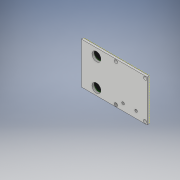
# Autodesk Inventor part: Печатная плата принимающая ось Z
Saved by Autodesk Inventor 2019 (Build 230136000, 136)
## iProperties
Created: 2019-08-27
Part Number: Печатная плата принимающая ось Z
Material: Типовые
Document SubType Name: Modeling
Designer: Петров Иван
Density: 1 g/cm^3
Appearance: По умолчанию
Autodesk Inventor part; units mm, degrees
(part 1 of 3)
ref_plane "YZ Plane" through (0, 0, 0) normal (1, 0, 0) x (0, 1, 0)
ref_plane "XZ Plane" through (0, 0, 0) normal (0, 1, 0) x (-1, 0, 0)
ref_plane "XY Plane" through (0, 0, 0) normal (0, 0, 1) x (1, 0, 0)
sketch "Эскиз1" plane through (0, 0, 0) normal (0, 0, 1) x (1, 0, 0)
  arc A0 (33.9725, 26.67) -> (33.3375, 26.67) centre (33.655, 26.67) ccw
  line L0 (27.051, 13.335) -> (30.988, 13.335)
  arc A1 (30.988, 13.0175) -> (30.988, 13.6525) centre (30.988, 13.335) ccw
  arc A2 (27.051, 13.6525) -> (27.051, 13.0175) centre (27.051, 13.335) ccw
  arc A3 (33.3375, 22.479) -> (33.9725, 22.479) centre (33.655, 22.479) ccw
  line L1 (33.655, 26.67) -> (33.655, 22.479)
  arc A4 (29.6525, 6.225) -> (30.2875, 6.225) centre (29.97, 6.225) ccw
  line L2 (29.97, 7.38) -> (29.97, 6.225)
  arc A5 (44.9285, 12.5435) -> (44.4795, 12.0945) centre (44.704, 12.319) ccw
  arc A6 (44.6575, 11.9165) -> (45.1065, 12.3655) centre (44.882, 12.141) ccw
  line L3 (44.704, 12.319) -> (44.882, 12.141)
  arc A7 (45.0215, 13.208) -> (44.3865, 13.208) centre (44.704, 13.208) ccw
  arc A8 (44.3865, 12.319) -> (45.0215, 12.319) centre (44.704, 12.319) ccw
  line L4 (44.704, 13.208) -> (44.704, 12.319)
  arc A9 (37.8165, 34.5145) -> (37.3675, 34.0655) centre (37.592, 34.29) ccw
  arc A10 (41.1775, 30.2555) -> (41.6265, 30.7045) centre (41.402, 30.48) ccw
  line L5 (37.592, 34.29) -> (41.402, 30.48)
  arc A11 (36.83, 34.6075) -> (36.83, 33.9725) centre (36.83, 34.29) ccw
  arc A12 (37.592, 33.9725) -> (37.592, 34.6075) centre (37.592, 34.29) ccw
  line L6 (36.83, 34.29) -> (37.592, 34.29)
  arc A13 (32.3555, 34.0655) -> (31.9065, 34.5145) centre (32.131, 34.29) ccw
  arc A14 (29.3665, 31.9745) -> (29.8155, 31.5255) centre (29.591, 31.75) ccw
  line L7 (32.131, 34.29) -> (29.591, 31.75)
  arc A15 (36.83, 33.9725) -> (36.83, 34.6075) centre (36.83, 34.29) ccw
  arc A16 (32.131, 34.6075) -> (32.131, 33.9725) centre (32.131, 34.29) ccw
  line L8 (36.83, 34.29) -> (32.131, 34.29)
  arc A17 (29.591, 31.4325) -> (29.591, 32.0675) centre (29.591, 31.75) ccw
  arc A18 (26.67, 32.0675) -> (26.67, 31.4325) centre (26.67, 31.75) ccw
  line L9 (29.591, 31.75) -> (26.67, 31.75)
  arc A19 (40.4155, 22.1955) -> (40.8645, 21.7465) centre (40.64, 21.971) ccw
  arc A20 (41.6265, 22.5085) -> (41.1775, 22.9575) centre (41.402, 22.733) ccw
  line L10 (40.64, 21.971) -> (41.402, 22.733)
  arc A21 (41.7195, 22.733) -> (41.0845, 22.733) centre (41.402, 22.733) ccw
  line L11 (26.289, 14.097) -> (27.051, 13.335)
  arc A22 (24.638, 24.8285) -> (24.638, 24.1935) centre (24.638, 24.511) ccw
  arc A23 (38.1, 24.1935) -> (38.1, 24.8285) centre (38.1, 24.511) ccw
  line L12 (24.638, 24.511) -> (38.1, 24.511)
  arc A24 (22.0005, 22.3225) -> (22.4495, 21.8735) centre (22.225, 22.098) ccw
  arc A25 (24.8625, 24.2865) -> (24.4135, 24.7355) centre (24.638, 24.511) ccw
  line L13 (22.225, 22.098) -> (24.638, 24.511)
  arc A26 (21.0185, 20.574) -> (20.3835, 20.574) centre (20.701, 20.574) ccw
  arc A27 (20.3835, 15.24) -> (21.0185, 15.24) centre (20.701, 15.24) ccw
  line L14 (20.701, 20.574) -> (20.701, 15.24)
  arc A28 (22.4495, 21.8735) -> (22.0005, 22.3225) centre (22.225, 22.098) ccw
  arc A29 (20.4765, 20.7985) -> (20.9255, 20.3495) centre (20.701, 20.574) ccw
  line L15 (22.225, 22.098) -> (20.701, 20.574)
  line L16 (22.225, 19.558) -> (26.035, 16.637)
  arc A30 (19.0205, 12.9245) -> (18.5715, 12.4755) centre (18.796, 12.7) ccw
  arc A31 (20.0955, 10.9515) -> (20.5445, 11.4005) centre (20.32, 11.176) ccw
  line L17 (18.796, 12.7) -> (20.32, 11.176)
  arc A32 (19.1135, 21.971) -> (18.4785, 21.971) centre (18.796, 21.971) ccw
  arc A33 (18.4785, 12.7) -> (19.1135, 12.7) centre (18.796, 12.7) ccw
  line L18 (18.796, 21.971) -> (18.796, 12.7)
  arc A34 (20.32, 11.3665) -> (20.32, 10.7315) centre (20.32, 11.049) ccw
  arc A35 (24.261, 10.7315) -> (24.261, 11.3665) centre (24.261, 11.049) ccw
  line L19 (20.32, 11.049) -> (24.261, 11.049)
  arc A36 (27.7055, 7.1555) -> (28.1545, 7.6045) centre (27.93, 7.38) ccw
  arc A37 (24.4855, 11.2735) -> (24.0365, 10.8245) centre (24.261, 11.049) ccw
  line L20 (27.93, 7.38) -> (24.261, 11.049)
  arc A38 (33.9725, 22.479) -> (33.3375, 22.479) centre (33.655, 22.479) ccw
  arc A39 (33.3375, 19.304) -> (33.9725, 19.304) centre (33.655, 19.304) ccw
  line L21 (33.655, 22.479) -> (33.655, 19.304)
  arc A40 (21.59, 26.9875) -> (21.59, 26.3525) centre (21.59, 26.67) ccw
  arc A41 (33.655, 26.3525) -> (33.655, 26.9875) centre (33.655, 26.67) ccw
  line L22 (21.59, 26.67) -> (33.655, 26.67)
  arc A42 (21.59, 26.3525) -> (20.955, 26.3525) centre (21.2725, 26.3525) ccw
  arc A43 (20.955, 24.4475) -> (21.59, 24.4475) centre (21.2725, 24.4475) ccw
  line L23 (21.2725, 26.3525) -> (21.2725, 24.4475)
  arc A44 (21.8145, 26.4455) -> (21.3655, 26.8945) centre (21.59, 26.67) ccw
  arc A45 (21.048, 26.577) -> (21.497, 26.128) centre (21.2725, 26.3525) ccw
  line L24 (21.59, 26.67) -> (21.2725, 26.3525)
  arc A46 (18.5715, 22.1955) -> (19.0205, 21.7465) centre (18.796, 21.971) ccw
  arc A47 (21.497, 24.223) -> (21.048, 24.672) centre (21.2725, 24.4475) ccw
  line L25 (18.796, 21.971) -> (21.2725, 24.4475)
  arc A48 (37.7485, 19.5285) -> (38.1975, 19.0795) centre (37.973, 19.304) ccw
  arc A49 (38.3245, 19.2065) -> (37.8755, 19.6555) centre (38.1, 19.431) ccw
  line L26 (37.973, 19.304) -> (38.1, 19.431)
  arc A50 (33.655, 19.6215) -> (33.655, 18.9865) centre (33.655, 19.304) ccw
  arc A51 (41.0845, 21.209) -> (41.7195, 21.209) centre (41.402, 21.209) ccw
  line L27 (41.402, 22.733) -> (41.402, 21.209)
  arc A52 (41.7195, 30.48) -> (41.0845, 30.48) centre (41.402, 30.48) ccw
  arc A53 (41.0845, 22.733) -> (41.7195, 22.733) centre (41.402, 22.733) ccw
  line L28 (41.402, 30.48) -> (41.402, 22.733)
  arc A54 (41.6265, 15.9725) -> (41.1775, 15.5235) centre (41.402, 15.748) ccw
  arc A55 (41.6855, 15.0155) -> (42.1345, 15.4645) centre (41.91, 15.24) ccw
  line L29 (41.402, 15.748) -> (41.91, 15.24)
  arc A56 (41.7195, 15.875) -> (41.0845, 15.875) centre (41.402, 15.875) ccw
  arc A57 (41.0845, 15.748) -> (41.7195, 15.748) centre (41.402, 15.748) ccw
  line L30 (41.402, 15.875) -> (41.402, 15.748)
  arc A58 (41.6265, 15.6505) -> (41.1775, 16.0995) centre (41.402, 15.875) ccw
  arc A59 (40.5425, 15.4645) -> (40.9915, 15.0155) centre (40.767, 15.24) ccw
  line L31 (41.402, 15.875) -> (40.767, 15.24)
  arc A60 (41.7195, 21.209) -> (41.0845, 21.209) centre (41.402, 21.209) ccw
  arc A61 (41.0845, 15.875) -> (41.7195, 15.875) centre (41.402, 15.875) ccw
  line L32 (41.402, 21.209) -> (41.402, 15.875)
  arc A62 (40.8645, 22.1955) -> (40.4155, 21.7465) centre (40.64, 21.971) ccw
  arc A63 (41.1775, 20.9845) -> (41.6265, 21.4335) centre (41.402, 21.209) ccw
  line L33 (40.64, 21.971) -> (41.402, 21.209)
  arc A64 (38.1, 22.2885) -> (38.1, 21.6535) centre (38.1, 21.971) ccw
  arc A65 (40.64, 21.6535) -> (40.64, 22.2885) centre (40.64, 21.971) ccw
  line L34 (38.1, 21.971) -> (40.64, 21.971)
  arc A66 (42.8965, 15.4645) -> (42.4475, 15.0155) centre (42.672, 15.24) ccw
  arc A67 (44.4795, 12.9835) -> (44.9285, 13.4325) centre (44.704, 13.208) ccw
  line L35 (42.672, 15.24) -> (44.704, 13.208)
  arc A68 (41.91, 15.5575) -> (41.91, 14.9225) centre (41.91, 15.24) ccw
  arc A69 (42.672, 14.9225) -> (42.672, 15.5575) centre (42.672, 15.24) ccw
  line L36 (41.91, 15.24) -> (42.672, 15.24)
  arc A70 (40.767, 15.5575) -> (40.767, 14.9225) centre (40.767, 15.24) ccw
  arc A71 (41.91, 14.9225) -> (41.91, 15.5575) centre (41.91, 15.24) ccw
  line L37 (40.767, 15.24) -> (41.91, 15.24)
  arc A72 (35.052, 15.5575) -> (35.052, 14.9225) centre (35.052, 15.24) ccw
  arc A73 (40.767, 14.9225) -> (40.767, 15.5575) centre (40.767, 15.24) ccw
  line L38 (35.052, 15.24) -> (40.767, 15.24)
  arc A74 (33.8795, 16.8615) -> (33.4305, 16.4125) centre (33.655, 16.637) ccw
  arc A75 (34.8275, 15.0155) -> (35.2765, 15.4645) centre (35.052, 15.24) ccw
  line L39 (33.655, 16.637) -> (35.052, 15.24)
  arc A76 (31.623, 16.9545) -> (31.623, 16.3195) centre (31.623, 16.637) ccw
  arc A77 (33.655, 16.3195) -> (33.655, 16.9545) centre (33.655, 16.637) ccw
  line L40 (31.623, 16.637) -> (33.655, 16.637)
  arc A78 (31.2125, 17.4965) -> (30.7635, 17.0475) centre (30.988, 17.272) ccw
  arc A79 (31.3985, 16.4125) -> (31.8475, 16.8615) centre (31.623, 16.637) ccw
  line L41 (30.988, 17.272) -> (31.623, 16.637)
  arc A80 (31.3055, 17.399) -> (30.6705, 17.399) centre (30.988, 17.399) ccw
  arc A81 (30.6705, 17.272) -> (31.3055, 17.272) centre (30.988, 17.272) ccw
  line L42 (30.988, 17.399) -> (30.988, 17.272)
  arc A82 (29.4345, 19.4015) -> (28.9855, 18.9525) centre (29.21, 19.177) ccw
  arc A83 (30.7635, 17.1745) -> (31.2125, 17.6235) centre (30.988, 17.399) ccw
  line L43 (29.21, 19.177) -> (30.988, 17.399)
  arc A84 (37.0005, 10.1445) -> (37.4495, 9.6955) centre (37.225, 9.92) ccw
  arc A85 (26.162, 19.4945) -> (26.162, 18.8595) centre (26.162, 19.177) ccw
  arc A86 (29.21, 18.8595) -> (29.21, 19.4945) centre (29.21, 19.177) ccw
  line L44 (26.162, 19.177) -> (29.21, 19.177)
  arc A87 (26.2595, 19.5285) -> (25.8105, 19.0795) centre (26.035, 19.304) ccw
  arc A88 (25.9375, 18.9525) -> (26.3865, 19.4015) centre (26.162, 19.177) ccw
  line L45 (26.035, 19.304) -> (26.162, 19.177)
  arc A89 (27.5175, 16.8615) -> (27.0685, 16.4125) centre (27.293, 16.637) ccw
  arc A90 (28.7255, 14.7555) -> (29.1745, 15.2045) centre (28.95, 14.98) ccw
  line L46 (27.293, 16.637) -> (28.95, 14.98)
  arc A91 (26.035, 16.9545) -> (26.035, 16.3195) centre (26.035, 16.637) ccw
  arc A92 (27.293, 16.3195) -> (27.293, 16.9545) centre (27.293, 16.637) ccw
  line L47 (26.035, 16.637) -> (27.293, 16.637)
  arc A93 (29.2675, 14.98) -> (28.6325, 14.98) centre (28.95, 14.98) ccw
  arc A94 (28.6325, 9.92) -> (29.2675, 9.92) centre (28.95, 9.92) ccw
  line L48 (28.95, 14.98) -> (28.95, 9.92)
  arc A95 (24.892, 22.5425) -> (24.892, 21.9075) centre (24.892, 22.225) ccw
  arc A96 (30.988, 21.9075) -> (30.988, 22.5425) centre (30.988, 22.225) ccw
  line L49 (24.892, 22.225) -> (30.988, 22.225)
  arc A97 (22.0005, 19.7825) -> (22.4495, 19.3335) centre (22.225, 19.558) ccw
  arc A98 (25.1165, 22.0005) -> (24.6675, 22.4495) centre (24.892, 22.225) ccw
  line L50 (22.225, 19.558) -> (24.892, 22.225)
  arc A99 (22.4182, 19.81) -> (22.0318, 19.306) centre (22.225, 19.558) ccw
  arc A100 (25.8418, 16.385) -> (26.2282, 16.889) centre (26.035, 16.637) ccw
  arc A101 (20.6375, 11.176) -> (20.0025, 11.176) centre (20.32, 11.176) ccw
  arc A102 (20.0025, 11.049) -> (20.6375, 11.049) centre (20.32, 11.049) ccw
  line L51 (20.32, 11.176) -> (20.32, 11.049)
  arc A103 (37.973, 18.9865) -> (37.973, 19.6215) centre (37.973, 19.304) ccw
  line L52 (33.655, 19.304) -> (37.973, 19.304)
  arc A104 (39.878, 7.8105) -> (39.878, 8.4455) centre (39.878, 8.128) ccw
  arc A105 (32.758, 8.4455) -> (32.758, 7.8105) centre (32.758, 8.128) ccw
  line L53 (39.878, 8.128) -> (32.758, 8.128)
  arc A106 (42.1345, 9.9355) -> (41.6855, 10.3845) centre (41.91, 10.16) ccw
  arc A107 (39.6535, 8.3525) -> (40.1025, 7.9035) centre (39.878, 8.128) ccw
  line L54 (41.91, 10.16) -> (39.878, 8.128)
  arc A108 (42.2275, 12.065) -> (41.5925, 12.065) centre (41.91, 12.065) ccw
  arc A109 (41.5925, 10.16) -> (42.2275, 10.16) centre (41.91, 10.16) ccw
  line L55 (41.91, 12.065) -> (41.91, 10.16)
  arc A110 (42.3885, 12.0945) -> (41.9395, 12.5435) centre (42.164, 12.319) ccw
  arc A111 (41.6855, 12.2895) -> (42.1345, 11.8405) centre (41.91, 12.065) ccw
  line L56 (42.164, 12.319) -> (41.91, 12.065)
  arc A112 (32.9825, 7.9035) -> (32.5335, 8.3525) centre (32.758, 8.128) ccw
  arc A113 (31.7855, 7.6045) -> (32.2345, 7.1555) centre (32.01, 7.38) ccw
  line L57 (32.758, 8.128) -> (32.01, 7.38)
  arc A114 (31.2125, 10.1465) -> (30.7635, 9.6975) centre (30.988, 9.922) ccw
  arc A115 (30.7655, 9.6955) -> (31.2145, 10.1445) centre (30.99, 9.92) ccw
  line L58 (30.988, 9.922) -> (30.99, 9.92)
  arc A116 (31.3055, 13.335) -> (30.6705, 13.335) centre (30.988, 13.335) ccw
  arc A117 (30.6705, 9.922) -> (31.3055, 9.922) centre (30.988, 9.922) ccw
  line L59 (30.988, 13.335) -> (30.988, 9.922)
  arc A118 (21.844, 14.4145) -> (21.844, 13.7795) centre (21.844, 14.097) ccw
  arc A119 (26.289, 13.7795) -> (26.289, 14.4145) centre (26.289, 14.097) ccw
  line L60 (21.844, 14.097) -> (26.289, 14.097)
  arc A120 (20.9255, 15.4645) -> (20.4765, 15.0155) centre (20.701, 15.24) ccw
  arc A121 (21.6195, 13.8725) -> (22.0685, 14.3215) centre (21.844, 14.097) ccw
  line L61 (20.701, 15.24) -> (21.844, 14.097)
  arc A122 (26.5135, 14.3215) -> (26.0645, 13.8725) centre (26.289, 14.097) ccw
  arc A123 (26.8265, 13.1105) -> (27.2755, 13.5595) centre (27.051, 13.335) ccw
  arc A124 (39.8485, 12.0945) -> (39.3995, 12.5435) centre (39.624, 12.319) ccw
  line L62 (37.225, 9.92) -> (39.624, 12.319)
  arc A125 (33.03, 10.2375) -> (33.03, 9.6025) centre (33.03, 9.92) ccw
  arc A126 (37.225, 9.6025) -> (37.225, 10.2375) centre (37.225, 9.92) ccw
  line L63 (33.03, 9.92) -> (37.225, 9.92)
  arc A127 (21.59, 34.6075) -> (21.59, 33.9725) centre (21.59, 34.29) ccw
  arc A128 (26.67, 33.9725) -> (26.67, 34.6075) centre (26.67, 34.29) ccw
  line L64 (21.59, 34.29) -> (26.67, 34.29)
  arc A129 (34.7005, 30.0695) -> (35.1495, 29.6205) centre (34.925, 29.845) ccw
  arc A130 (37.0545, 31.5255) -> (36.6055, 31.9745) centre (36.83, 31.75) ccw
  line L65 (34.925, 29.845) -> (36.83, 31.75)
  arc A131 (30.988, 30.1625) -> (30.988, 29.5275) centre (30.988, 29.845) ccw
  arc A132 (34.925, 29.5275) -> (34.925, 30.1625) centre (34.925, 29.845) ccw
  line L66 (30.988, 29.845) -> (34.925, 29.845)
  arc A133 (45.1065, 7.1925) -> (44.6575, 7.6415) centre (44.882, 7.417) ccw
  arc A134 (39.4895, 2.4735) -> (39.9385, 2.0245) centre (39.714, 2.249) ccw
  line L67 (44.882, 7.417) -> (39.714, 2.249)
  arc A135 (45.1995, 12.141) -> (44.5645, 12.141) centre (44.882, 12.141) ccw
  arc A136 (44.5645, 7.417) -> (45.1995, 7.417) centre (44.882, 7.417) ccw
  line L68 (44.882, 12.141) -> (44.882, 7.417)
  arc A137 (30.1945, 6.4495) -> (29.7455, 6.0005) centre (29.97, 6.225) ccw
  arc A138 (33.7215, 2.0245) -> (34.1705, 2.4735) centre (33.946, 2.249) ccw
  line L69 (29.97, 6.225) -> (33.946, 2.249)
  arc A139 (39.714, 1.9315) -> (39.714, 2.5665) centre (39.714, 2.249) ccw
  arc A140 (33.946, 2.5665) -> (33.946, 1.9315) centre (33.946, 2.249) ccw
  line L70 (39.714, 2.249) -> (33.946, 2.249)
  arc A141 (30.2875, 7.38) -> (29.6525, 7.38) centre (29.97, 7.38) ccw
  line L71 (46.533, -1.143) -> (46.533, 36.947)
  line L72 (46.533, 36.947) -> (-13.871, 36.947)
  line L73 (-13.871, 36.947) -> (-13.871, -1.143)
  circle A142 centre (17.907, 34.925) radius 1.5
  circle A143 centre (17.907, 0.762) radius 1.5
  circle A144 centre (44.577, 0.762) radius 1.5
  circle A145 centre (44.704, 35.052) radius 1.5
  circle A146 centre (0, 30) radius 4.1
  circle A147 centre (0, 5) radius 4.1
  circle A148 centre (24.48, 5.08) radius 1.18
  line L74 (-13.871, -1.143) -> (46.533, -1.143)
  circle A149 centre (36.48, 5.08) radius 1.18
  arc A150 (39.8159, 21.3614) -> (39.8159, 21.4122) centre (39.8159, 21.3868) ccw
  arc A151 (39.1668, 21.6464) -> (39.4264, 21.3868) centre (39.4264, 21.6464) ccw
  arc A152 (39.1922, 21.6464) -> (39.1414, 21.6464) centre (39.1668, 21.6464) ccw
  arc A153 (39.4264, 21.3614) -> (39.4264, 21.4122) centre (39.4264, 21.3868) ccw
  line L75 (39.1668, 21.6464) -> (39.1668, 22.2956)
  arc A154 (39.1922, 22.2956) -> (39.1414, 22.2956) centre (39.1668, 22.2956) ccw
  arc A155 (39.1414, 21.6464) -> (39.1922, 21.6464) centre (39.1668, 21.6464) ccw
  arc A156 (39.4264, 22.5552) -> (39.1668, 22.2956) centre (39.4264, 22.2956) ccw
  arc A157 (39.4264, 22.5298) -> (39.4264, 22.5806) centre (39.4264, 22.5552) ccw
  arc A158 (39.1414, 22.2956) -> (39.1922, 22.2956) centre (39.1668, 22.2956) ccw
  line L76 (24.765, 30.48) -> (28.575, 30.48)
  arc A159 (28.575, 30.4292) -> (28.575, 30.5308) centre (28.575, 30.48) ccw
  arc A160 (24.765, 30.5308) -> (24.765, 30.4292) centre (24.765, 30.48) ccw
  arc A161 (28.575, 30.48) -> (24.765, 30.48) centre (26.67, 33.02) ccw
  line L77 (39.4264, 22.5552) -> (39.8159, 22.5552)
  arc A162 (39.8159, 22.5298) -> (39.8159, 22.5806) centre (39.8159, 22.5552) ccw
  arc A163 (39.4264, 22.5806) -> (39.4264, 22.5298) centre (39.4264, 22.5552) ccw
  line L78 (40.386, 21.3868) -> (40.386, 22.5552)
  arc A164 (40.4114, 22.5552) -> (40.3606, 22.5552) centre (40.386, 22.5552) ccw
  arc A165 (40.3606, 21.3868) -> (40.4114, 21.3868) centre (40.386, 21.3868) ccw
  line L79 (40.386, 22.5552) -> (41.0351, 21.3868)
  arc A166 (41.0129, 21.3745) -> (41.0573, 21.3991) centre (41.0351, 21.3868) ccw
  arc A167 (40.4082, 22.5675) -> (40.3638, 22.5429) centre (40.386, 22.5552) ccw
  line L80 (41.0351, 21.3868) -> (41.0351, 22.5552)
  arc A168 (41.0605, 22.5552) -> (41.0097, 22.5552) centre (41.0351, 22.5552) ccw
  arc A169 (41.0097, 21.3868) -> (41.0605, 21.3868) centre (41.0351, 21.3868) ccw
  line L81 (41.6052, 21.3868) -> (41.6052, 22.5552)
  arc A170 (41.6306, 22.5552) -> (41.5798, 22.5552) centre (41.6052, 22.5552) ccw
  arc A171 (41.5798, 21.3868) -> (41.6306, 21.3868) centre (41.6052, 21.3868) ccw
  line L82 (41.6052, 22.5552) -> (41.9297, 22.5552)
  arc A172 (41.9297, 22.5298) -> (41.9297, 22.5806) centre (41.9297, 22.5552) ccw
  arc A173 (41.6052, 22.5806) -> (41.6052, 22.5298) centre (41.6052, 22.5552) ccw
  arc A174 (42.2543, 22.2306) -> (41.9297, 22.5552) centre (41.9297, 22.2306) ccw
  arc A175 (42.2289, 22.2306) -> (42.2797, 22.2306) centre (42.2543, 22.2306) ccw
  arc A176 (41.9297, 22.5806) -> (41.9297, 22.5298) centre (41.9297, 22.5552) ccw
  line L83 (42.2543, 22.2306) -> (42.2543, 21.7114)
  arc A177 (42.2289, 21.7114) -> (42.2797, 21.7114) centre (42.2543, 21.7114) ccw
  arc A178 (42.2797, 22.2306) -> (42.2289, 22.2306) centre (42.2543, 22.2306) ccw
  arc A179 (41.9297, 21.3868) -> (42.2543, 21.7114) centre (41.9297, 21.7114) ccw
  arc A180 (41.9297, 21.4122) -> (41.9297, 21.3614) centre (41.9297, 21.3868) ccw
  arc A181 (42.2797, 21.7114) -> (42.2289, 21.7114) centre (42.2543, 21.7114) ccw
  line L84 (41.9297, 21.3868) -> (41.6052, 21.3868)
  arc A182 (41.6052, 21.4122) -> (41.6052, 21.3614) centre (41.6052, 21.3868) ccw
  arc A183 (41.9297, 21.3614) -> (41.9297, 21.4122) centre (41.9297, 21.3868) ccw
  arc A184 (26.67, 30.48) -> (26.67, 35.56) centre (26.67, 33.02) ccw
  arc A185 (26.67, 35.56) -> (26.67, 30.48) centre (26.67, 33.02) ccw
  line L85 (39.2938, 18.8468) -> (39.2938, 20.0152)
  arc A186 (39.3192, 20.0152) -> (39.2684, 20.0152) centre (39.2938, 20.0152) ccw
  arc A187 (39.2684, 18.8468) -> (39.3192, 18.8468) centre (39.2938, 18.8468) ccw
  line L86 (39.2938, 20.0152) -> (39.6184, 20.0152)
  arc A188 (39.6184, 19.9898) -> (39.6184, 20.0406) centre (39.6184, 20.0152) ccw
  arc A189 (39.2938, 20.0406) -> (39.2938, 19.9898) centre (39.2938, 20.0152) ccw
  arc A190 (39.9429, 19.6906) -> (39.6184, 20.0152) centre (39.6183, 19.6906) ccw
  arc A191 (39.9175, 19.6906) -> (39.9683, 19.6906) centre (39.9429, 19.6906) ccw
  arc A192 (39.6184, 20.0406) -> (39.6184, 19.9898) centre (39.6184, 20.0152) ccw
  line L87 (39.9429, 19.6906) -> (39.9429, 19.1714)
  line L88 (38.735, 35.56) -> (34.925, 35.56)
  arc A193 (34.925, 35.6108) -> (34.925, 35.5092) centre (34.925, 35.56) ccw
  arc A194 (38.735, 35.5092) -> (38.735, 35.6108) centre (38.735, 35.56) ccw
  arc A195 (34.925, 35.56) -> (38.735, 35.56) centre (36.83, 33.02) ccw
  arc A196 (39.9175, 19.1714) -> (39.9683, 19.1714) centre (39.9429, 19.1714) ccw
  arc A197 (39.9683, 19.6906) -> (39.9175, 19.6906) centre (39.9429, 19.6906) ccw
  arc A198 (39.6184, 18.8468) -> (39.9429, 19.1714) centre (39.6183, 19.1714) ccw
  arc A199 (39.6184, 18.8722) -> (39.6184, 18.8214) centre (39.6184, 18.8468) ccw
  arc A200 (39.9683, 19.1714) -> (39.9175, 19.1714) centre (39.9429, 19.1714) ccw
  line L89 (39.6184, 18.8468) -> (39.2938, 18.8468)
  arc A201 (39.2938, 18.8722) -> (39.2938, 18.8214) centre (39.2938, 18.8468) ccw
  arc A202 (39.6184, 18.8214) -> (39.6184, 18.8722) centre (39.6184, 18.8468) ccw
  line L90 (40.4749, 19.1714) -> (40.4749, 19.6906)
  arc A203 (40.5003, 19.6906) -> (40.4495, 19.6906) centre (40.4749, 19.6906) ccw
  arc A204 (41.124, 19.6906) -> (40.4749, 19.6906) centre (40.7995, 19.6906) ccw
  arc A205 (41.0986, 19.6906) -> (41.1494, 19.6906) centre (41.124, 19.6906) ccw
  arc A206 (40.4495, 19.6906) -> (40.5003, 19.6906) centre (40.4749, 19.6906) ccw
  line L91 (41.124, 19.6906) -> (41.124, 19.1714)
  arc A207 (41.0986, 19.1714) -> (41.1494, 19.1714) centre (41.124, 19.1714) ccw
  arc A208 (41.1494, 19.6906) -> (41.0986, 19.6906) centre (41.124, 19.6906) ccw
  arc A209 (40.4749, 19.1714) -> (41.124, 19.1714) centre (40.7995, 19.1714) ccw
  arc A210 (40.5003, 19.1714) -> (40.4495, 19.1714) centre (40.4749, 19.1714) ccw
  arc A211 (41.1494, 19.1714) -> (41.0986, 19.1714) centre (41.124, 19.1714) ccw
  line L92 (39.2938, 16.5608) -> (39.6833, 17.7292)
  arc A212 (39.7074, 17.7212) -> (39.6592, 17.7372) centre (39.6833, 17.7292) ccw
  arc A213 (39.2697, 16.5688) -> (39.3179, 16.5528) centre (39.2938, 16.5608) ccw
  line L93 (39.6833, 17.7292) -> (40.0727, 16.5608)
  arc A214 (40.0486, 16.5528) -> (40.0968, 16.5688) centre (40.0727, 16.5608) ccw
  arc A215 (39.7074, 17.7372) -> (39.6592, 17.7212) centre (39.6833, 17.7292) ccw
  line L94 (39.9754, 16.8529) -> (39.3912, 16.8529)
  arc A216 (39.3912, 16.8783) -> (39.3912, 16.8275) centre (39.3912, 16.8529) ccw
  arc A217 (39.9754, 16.8275) -> (39.9754, 16.8783) centre (39.9754, 16.8529) ccw
  line L95 (40.5017, 16.8854) -> (40.5017, 17.4046)
  arc A218 (40.5271, 17.4046) -> (40.4763, 17.4046) centre (40.5017, 17.4046) ccw
  arc A219 (40.4763, 16.8854) -> (40.5271, 16.8854) centre (40.5017, 16.8854) ccw
  arc A220 (41.1508, 17.4046) -> (40.5017, 17.4046) centre (40.8263, 17.4046) ccw
  arc A221 (41.1254, 17.4046) -> (41.1762, 17.4046) centre (41.1508, 17.4046) ccw
  arc A222 (40.4763, 17.4046) -> (40.5271, 17.4046) centre (40.5017, 17.4046) ccw
  line L96 (41.1508, 17.4046) -> (41.1508, 16.8854)
  arc A223 (41.1254, 16.8854) -> (41.1762, 16.8854) centre (41.1508, 16.8854) ccw
  arc A224 (36.83, 30.48) -> (36.83, 35.56) centre (36.83, 33.02) ccw
  arc A225 (36.83, 35.56) -> (36.83, 30.48) centre (36.83, 33.02) ccw
  arc A226 (41.1762, 17.4046) -> (41.1254, 17.4046) centre (41.1508, 17.4046) ccw
  line L97 (45.974, 13.589) -> (45.974, 11.684)
  arc A227 (45.9423, 11.684) -> (46.0058, 11.684) centre (45.9741, 11.684) ccw
  arc A228 (46.0058, 13.589) -> (45.9423, 13.589) centre (45.9741, 13.589) ccw
  line L98 (45.974, 11.684) -> (45.339, 11.049)
  arc A229 (45.3165, 11.0715) -> (45.3615, 11.0265) centre (45.339, 11.049) ccw
  arc A230 (45.9965, 11.6615) -> (45.9515, 11.7065) centre (45.974, 11.684) ccw
  line L99 (45.339, 11.049) -> (44.069, 11.049)
  arc A231 (44.069, 11.0808) -> (44.069, 11.0173) centre (44.069, 11.0491) ccw
  arc A232 (45.339, 11.0173) -> (45.339, 11.0808) centre (45.339, 11.0491) ccw
  line L100 (44.069, 11.049) -> (43.434, 11.684)
  arc A233 (43.4565, 11.7065) -> (43.4115, 11.6615) centre (43.434, 11.684) ccw
  arc A234 (44.0465, 11.0265) -> (44.0915, 11.0715) centre (44.069, 11.049) ccw
  line L101 (43.434, 11.684) -> (42.799, 11.049)
  arc A235 (42.7765, 11.0715) -> (42.8215, 11.0265) centre (42.799, 11.049) ccw
  arc A236 (43.4565, 11.6615) -> (43.4115, 11.7065) centre (43.434, 11.684) ccw
  line L102 (42.799, 11.049) -> (41.529, 11.049)
  arc A237 (41.529, 11.0808) -> (41.529, 11.0173) centre (41.529, 11.0491) ccw
  arc A238 (42.799, 11.0173) -> (42.799, 11.0808) centre (42.799, 11.0491) ccw
  line L103 (41.529, 11.049) -> (40.894, 11.684)
  arc A239 (41.5065, 11.0265) -> (41.5515, 11.0715) centre (41.529, 11.049) ccw
  line L104 (40.894, 11.684) -> (40.259, 11.049)
  arc A240 (40.2365, 11.0715) -> (40.2815, 11.0265) centre (40.259, 11.049) ccw
  arc A241 (40.9165, 11.6615) -> (40.8715, 11.7065) centre (40.894, 11.684) ccw
  line L105 (40.259, 11.049) -> (38.989, 11.049)
  arc A242 (38.989, 11.0808) -> (38.989, 11.0173) centre (38.989, 11.0491) ccw
  arc A243 (40.259, 11.0173) -> (40.259, 11.0808) centre (40.259, 11.0491) ccw
  line L106 (38.989, 11.049) -> (38.354, 11.684)
  arc A244 (38.3765, 11.7065) -> (38.3315, 11.6615) centre (38.354, 11.684) ccw
  arc A245 (38.9665, 11.0265) -> (39.0115, 11.0715) centre (38.989, 11.049) ccw
  line L107 (38.354, 11.684) -> (38.354, 13.589)
  arc A246 (38.3858, 13.589) -> (38.3222, 13.589) centre (38.354, 13.589) ccw
  arc A247 (38.3222, 11.684) -> (38.3858, 11.684) centre (38.354, 11.684) ccw
  line L108 (38.354, 13.589) -> (45.974, 13.589)
  arc A248 (45.974, 13.5572) -> (45.974, 13.6208) centre (45.974, 13.589) ccw
  arc A249 (38.354, 13.6208) -> (38.354, 13.5572) centre (38.354, 13.589) ccw
  line L109 (37.719, 14.224) -> (46.609, 14.224)
  arc A250 (46.609, 14.1922) -> (46.609, 14.2558) centre (46.609, 14.224) ccw
  arc A251 (37.719, 14.2558) -> (37.719, 14.1922) centre (37.719, 14.224) ccw
  line L110 (46.609, 14.224) -> (46.609, 11.684)
  arc A252 (46.5772, 11.684) -> (46.6408, 11.684) centre (46.609, 11.684) ccw
  arc A253 (46.6408, 14.224) -> (46.5772, 14.224) centre (46.609, 14.224) ccw
  line L111 (46.609, 11.684) -> (45.974, 11.049)
  arc A254 (45.9515, 11.0715) -> (45.9965, 11.0265) centre (45.974, 11.049) ccw
  arc A255 (46.6315, 11.6615) -> (46.5865, 11.7065) centre (46.609, 11.684) ccw
  line L112 (45.974, 11.049) -> (37.719, 11.049)
  arc A256 (37.719, 11.0808) -> (37.719, 11.0173) centre (37.719, 11.0491) ccw
  arc A257 (45.974, 11.0173) -> (45.974, 11.0808) centre (45.974, 11.0491) ccw
  line L113 (37.719, 11.049) -> (37.719, 14.224)
  arc A258 (37.7508, 14.224) -> (37.6872, 14.224) centre (37.719, 14.224) ccw
  arc A259 (37.6872, 11.049) -> (37.7508, 11.049) centre (37.719, 11.049) ccw
  arc A260 (40.5017, 16.8854) -> (41.1508, 16.8854) centre (40.8263, 16.8854) ccw
  arc A261 (40.5271, 16.8854) -> (40.4763, 16.8854) centre (40.5017, 16.8854) ccw
  arc A262 (41.1762, 16.8854) -> (41.1254, 16.8854) centre (41.1508, 16.8854) ccw
  line L114 (19.685, 14.478) -> (24.765, 14.478)
  arc A263 (24.765, 14.4463) -> (24.765, 14.5098) centre (24.765, 14.478) ccw
  arc A264 (19.685, 14.5098) -> (19.685, 14.4463) centre (19.685, 14.478) ccw
  line L115 (24.765, 14.478) -> (24.765, 24.638)
  arc A265 (24.7967, 24.638) -> (24.7333, 24.638) centre (24.765, 24.638) ccw
  arc A266 (24.7333, 14.478) -> (24.7967, 14.478) centre (24.765, 14.478) ccw
  line L116 (24.765, 24.638) -> (19.685, 24.638)
  arc A267 (19.685, 24.6698) -> (19.685, 24.6063) centre (19.685, 24.6381) ccw
  arc A268 (24.765, 24.6063) -> (24.765, 24.6698) centre (24.765, 24.6381) ccw
  line L117 (19.685, 24.638) -> (19.685, 14.478)
  line L118 (24.38, 12.08) -> (36.58, 12.08)
  arc A269 (36.58, 12.0482) -> (36.58, 12.1118) centre (36.58, 12.08) ccw
  arc A270 (24.38, 12.1118) -> (24.38, 12.0482) centre (24.38, 12.08) ccw
  line L119 (36.58, 12.08) -> (36.58, -0.92)
  arc A271 (36.5482, -0.92) -> (36.6118, -0.92) centre (36.58, -0.92) ccw
  arc A272 (36.6118, 12.08) -> (36.5482, 12.08) centre (36.58, 12.08) ccw
  line L120 (36.58, -0.92) -> (24.38, -0.92)
  arc A273 (24.38, -0.8882) -> (24.38, -0.9518) centre (24.38, -0.92) ccw
  arc A274 (36.58, -0.9518) -> (36.58, -0.8882) centre (36.58, -0.92) ccw
  line L121 (24.38, -0.92) -> (24.38, 12.08)
  arc A275 (24.4118, 12.08) -> (24.3483, 12.08) centre (24.3801, 12.08) ccw
  arc A276 (24.3483, -0.92) -> (24.4118, -0.92) centre (24.3801, -0.92) ccw
  arc A277 (19.6533, 14.478) -> (19.7168, 14.478) centre (19.6851, 14.478) ccw
  arc A278 (19.7168, 24.638) -> (19.6533, 24.638) centre (19.6851, 24.638) ccw
  arc A279 (30.0101, 24.13) -> (29.9339, 24.13) centre (29.972, 24.13) ccw
  arc A280 (40.4495, 19.1714) -> (40.5003, 19.1714) centre (40.4749, 19.1714) ccw
  arc A281 (32.131, 15.621) -> (32.385, 15.875) centre (32.131, 15.875) ccw
  arc A282 (32.131, 15.6591) -> (32.131, 15.5829) centre (32.131, 15.621) ccw
  arc A283 (32.4231, 15.875) -> (32.3469, 15.875) centre (32.385, 15.875) ccw
  arc A284 (32.385, 17.399) -> (32.131, 17.653) centre (32.131, 17.399) ccw
  arc A285 (32.3469, 17.399) -> (32.4231, 17.399) centre (32.385, 17.399) ccw
  arc A286 (32.131, 17.6911) -> (32.131, 17.6149) centre (32.131, 17.653) ccw
  arc A287 (27.559, 17.653) -> (27.305, 17.399) centre (27.559, 17.399) ccw
  arc A288 (27.559, 17.6149) -> (27.559, 17.6911) centre (27.559, 17.653) ccw
  arc A289 (27.2669, 17.399) -> (27.3431, 17.399) centre (27.305, 17.399) ccw
  arc A290 (27.305, 15.875) -> (27.559, 15.621) centre (27.559, 15.875) ccw
  arc A291 (27.3431, 15.875) -> (27.2669, 15.875) centre (27.305, 15.875) ccw
  arc A292 (27.559, 15.5829) -> (27.559, 15.6591) centre (27.559, 15.621) ccw
  line L122 (32.385, 17.399) -> (32.385, 15.875)
  arc A293 (32.3469, 15.875) -> (32.4231, 15.875) centre (32.385, 15.875) ccw
  arc A294 (32.4231, 17.399) -> (32.3469, 17.399) centre (32.385, 17.399) ccw
  line L123 (32.131, 15.621) -> (31.75, 15.621)
  arc A295 (31.75, 15.6591) -> (31.75, 15.5829) centre (31.75, 15.621) ccw
  arc A296 (32.131, 15.5829) -> (32.131, 15.6591) centre (32.131, 15.621) ccw
  line L124 (31.623, 15.748) -> (31.75, 15.621)
  arc A297 (31.7231, 15.5941) -> (31.7769, 15.6479) centre (31.75, 15.621) ccw
  arc A298 (31.6499, 15.7749) -> (31.5961, 15.7211) centre (31.623, 15.748) ccw
  line L125 (32.131, 17.653) -> (31.75, 17.653)
  arc A299 (31.75, 17.6911) -> (31.75, 17.6149) centre (31.75, 17.653) ccw
  arc A300 (32.131, 17.6149) -> (32.131, 17.6911) centre (32.131, 17.653) ccw
  line L126 (31.623, 17.526) -> (31.75, 17.653)
  arc A301 (31.7769, 17.6261) -> (31.7231, 17.6799) centre (31.75, 17.653) ccw
  arc A302 (31.5961, 17.5529) -> (31.6499, 17.4991) centre (31.623, 17.526) ccw
  line L127 (28.067, 15.748) -> (27.94, 15.621)
  arc A303 (27.9131, 15.6479) -> (27.9669, 15.5941) centre (27.94, 15.621) ccw
  arc A304 (28.0939, 15.7211) -> (28.0401, 15.7749) centre (28.067, 15.748) ccw
  line L128 (28.067, 15.748) -> (31.623, 15.748)
  arc A305 (31.623, 15.7099) -> (31.623, 15.7861) centre (31.623, 15.748) ccw
  arc A306 (28.067, 15.7861) -> (28.067, 15.7099) centre (28.067, 15.748) ccw
  line L129 (28.067, 17.526) -> (27.94, 17.653)
  arc A307 (27.9669, 17.6799) -> (27.9131, 17.6261) centre (27.94, 17.653) ccw
  arc A308 (28.0401, 17.4991) -> (28.0939, 17.5529) centre (28.067, 17.526) ccw
  line L130 (28.067, 17.526) -> (31.623, 17.526)
  arc A309 (31.623, 17.4879) -> (31.623, 17.5641) centre (31.623, 17.526) ccw
  arc A310 (28.067, 17.5641) -> (28.067, 17.4879) centre (28.067, 17.526) ccw
  line L131 (27.559, 15.621) -> (27.94, 15.621)
  arc A311 (27.94, 15.5829) -> (27.94, 15.6591) centre (27.94, 15.621) ccw
  arc A312 (27.559, 15.6591) -> (27.559, 15.5829) centre (27.559, 15.621) ccw
  line L132 (27.559, 17.653) -> (27.94, 17.653)
  arc A313 (27.94, 17.6149) -> (27.94, 17.6911) centre (27.94, 17.653) ccw
  arc A314 (27.559, 17.6911) -> (27.559, 17.6149) centre (27.559, 17.653) ccw
  line L133 (27.305, 17.399) -> (27.305, 15.875)
  arc A315 (27.2669, 15.875) -> (27.3431, 15.875) centre (27.305, 15.875) ccw
  arc A316 (27.3431, 17.399) -> (27.2669, 17.399) centre (27.305, 17.399) ccw
  arc A317 (27.559, 20.32) -> (27.305, 20.066) centre (27.559, 20.066) ccw
  arc A318 (27.559, 20.2819) -> (27.559, 20.3581) centre (27.559, 20.32) ccw
  arc A319 (27.2669, 20.066) -> (27.3431, 20.066) centre (27.305, 20.066) ccw
  arc A320 (27.305, 18.542) -> (27.559, 18.288) centre (27.559, 18.542) ccw
  arc A321 (27.3431, 18.542) -> (27.2669, 18.542) centre (27.305, 18.542) ccw
  arc A322 (27.559, 18.2499) -> (27.559, 18.3261) centre (27.559, 18.288) ccw
  arc A323 (32.131, 18.288) -> (32.385, 18.542) centre (32.131, 18.542) ccw
  arc A324 (32.131, 18.3261) -> (32.131, 18.2499) centre (32.131, 18.288) ccw
  arc A325 (32.4231, 18.542) -> (32.3469, 18.542) centre (32.385, 18.542) ccw
  arc A326 (32.385, 20.066) -> (32.131, 20.32) centre (32.131, 20.066) ccw
  arc A327 (32.3469, 20.066) -> (32.4231, 20.066) centre (32.385, 20.066) ccw
  arc A328 (32.131, 20.3581) -> (32.131, 20.2819) centre (32.131, 20.32) ccw
  line L134 (27.305, 18.542) -> (27.305, 20.066)
  arc A329 (27.3431, 20.066) -> (27.2669, 20.066) centre (27.305, 20.066) ccw
  arc A330 (27.2669, 18.542) -> (27.3431, 18.542) centre (27.305, 18.542) ccw
  line L135 (27.559, 20.32) -> (27.94, 20.32)
  arc A331 (27.94, 20.2819) -> (27.94, 20.3581) centre (27.94, 20.32) ccw
  arc A332 (27.559, 20.3581) -> (27.559, 20.2819) centre (27.559, 20.32) ccw
  line L136 (28.067, 20.193) -> (27.94, 20.32)
  arc A333 (27.9669, 20.3469) -> (27.9131, 20.2931) centre (27.94, 20.32) ccw
  arc A334 (28.0401, 20.1661) -> (28.0939, 20.2199) centre (28.067, 20.193) ccw
  line L137 (27.559, 18.288) -> (27.94, 18.288)
  arc A335 (27.94, 18.2499) -> (27.94, 18.3261) centre (27.94, 18.288) ccw
  arc A336 (27.559, 18.3261) -> (27.559, 18.2499) centre (27.559, 18.288) ccw
  line L138 (28.067, 18.415) -> (27.94, 18.288)
  arc A337 (27.9131, 18.3149) -> (27.9669, 18.2611) centre (27.94, 18.288) ccw
  arc A338 (28.0939, 18.3881) -> (28.0401, 18.4419) centre (28.067, 18.415) ccw
  line L139 (31.623, 20.193) -> (31.75, 20.32)
  arc A339 (31.7769, 20.2931) -> (31.7231, 20.3469) centre (31.75, 20.32) ccw
  arc A340 (31.5961, 20.2199) -> (31.6499, 20.1661) centre (31.623, 20.193) ccw
  line L140 (31.623, 20.193) -> (28.067, 20.193)
  arc A341 (28.067, 20.2311) -> (28.067, 20.1549) centre (28.067, 20.193) ccw
  arc A342 (31.623, 20.1549) -> (31.623, 20.2311) centre (31.623, 20.193) ccw
  line L141 (31.623, 18.415) -> (31.75, 18.288)
  arc A343 (31.7231, 18.2611) -> (31.7769, 18.3149) centre (31.75, 18.288) ccw
  arc A344 (31.6499, 18.4419) -> (31.5961, 18.3881) centre (31.623, 18.415) ccw
  line L142 (31.623, 18.415) -> (28.067, 18.415)
  arc A345 (28.067, 18.4531) -> (28.067, 18.3769) centre (28.067, 18.415) ccw
  arc A346 (31.623, 18.3769) -> (31.623, 18.4531) centre (31.623, 18.415) ccw
  line L143 (32.131, 20.32) -> (31.75, 20.32)
  arc A347 (31.75, 20.3581) -> (31.75, 20.2819) centre (31.75, 20.32) ccw
  arc A348 (32.131, 20.2819) -> (32.131, 20.3581) centre (32.131, 20.32) ccw
  line L144 (32.131, 18.288) -> (31.75, 18.288)
  arc A349 (31.75, 18.3261) -> (31.75, 18.2499) centre (31.75, 18.288) ccw
  arc A350 (32.131, 18.2499) -> (32.131, 18.3261) centre (32.131, 18.288) ccw
  line L145 (32.385, 18.542) -> (32.385, 20.066)
  arc A351 (32.4231, 20.066) -> (32.3469, 20.066) centre (32.385, 20.066) ccw
  arc A352 (32.3469, 18.542) -> (32.4231, 18.542) centre (32.385, 18.542) ccw
  arc A353 (29.972, 23.749) -> (30.226, 23.495) centre (30.226, 23.749) ccw
  arc A354 (30.0101, 23.749) -> (29.9339, 23.749) centre (29.972, 23.749) ccw
  arc A355 (30.226, 23.4569) -> (30.226, 23.5331) centre (30.226, 23.495) ccw
  arc A356 (31.75, 23.495) -> (32.004, 23.749) centre (31.75, 23.749) ccw
  arc A357 (31.75, 23.5331) -> (31.75, 23.4569) centre (31.75, 23.495) ccw
  arc A358 (32.0421, 23.749) -> (31.9659, 23.749) centre (32.004, 23.749) ccw
  arc A359 (32.004, 28.321) -> (31.75, 28.575) centre (31.75, 28.321) ccw
  arc A360 (31.9659, 28.321) -> (32.0421, 28.321) centre (32.004, 28.321) ccw
  arc A361 (31.75, 28.6131) -> (31.75, 28.5369) centre (31.75, 28.575) ccw
  arc A362 (30.226, 28.575) -> (29.972, 28.321) centre (30.226, 28.321) ccw
  arc A363 (30.226, 28.5369) -> (30.226, 28.6131) centre (30.226, 28.575) ccw
  arc A364 (29.9339, 28.321) -> (30.0101, 28.321) centre (29.972, 28.321) ccw
  line L146 (31.75, 23.495) -> (30.226, 23.495)
  arc A365 (30.226, 23.5331) -> (30.226, 23.4569) centre (30.226, 23.495) ccw
  arc A366 (31.75, 23.4569) -> (31.75, 23.5331) centre (31.75, 23.495) ccw
  line L147 (29.972, 23.749) -> (29.972, 24.13)
  arc A367 (40.9165, 11.7065) -> (40.8715, 11.6615) centre (40.894, 11.684) ccw
  arc A368 (29.9339, 23.749) -> (30.0101, 23.749) centre (29.972, 23.749) ccw
  line L148 (30.099, 24.257) -> (29.972, 24.13)
  arc A369 (29.9451, 24.1569) -> (29.9989, 24.1031) centre (29.972, 24.13) ccw
  arc A370 (30.1259, 24.2301) -> (30.0721, 24.2839) centre (30.099, 24.257) ccw
  line L149 (32.004, 23.749) -> (32.004, 24.13)
  arc A371 (32.0421, 24.13) -> (31.9659, 24.13) centre (32.004, 24.13) ccw
  arc A372 (31.9659, 23.749) -> (32.0421, 23.749) centre (32.004, 23.749) ccw
  line L150 (31.877, 24.257) -> (32.004, 24.13)
  arc A373 (31.9771, 24.1031) -> (32.0309, 24.1569) centre (32.004, 24.13) ccw
  arc A374 (31.9039, 24.2839) -> (31.8501, 24.2301) centre (31.877, 24.257) ccw
  line L151 (30.099, 27.813) -> (29.972, 27.94)
  arc A375 (29.9989, 27.9669) -> (29.9451, 27.9131) centre (29.972, 27.94) ccw
  arc A376 (30.0721, 27.7861) -> (30.1259, 27.8399) centre (30.099, 27.813) ccw
  line L152 (30.099, 27.813) -> (30.099, 24.257)
  arc A377 (30.0609, 24.257) -> (30.1371, 24.257) centre (30.099, 24.257) ccw
  arc A378 (30.1371, 27.813) -> (30.0609, 27.813) centre (30.099, 27.813) ccw
  line L153 (31.877, 27.813) -> (32.004, 27.94)
  arc A379 (32.0309, 27.9131) -> (31.9771, 27.9669) centre (32.004, 27.94) ccw
  arc A380 (31.8501, 27.8399) -> (31.9039, 27.7861) centre (31.877, 27.813) ccw
  line L154 (31.877, 27.813) -> (31.877, 24.257)
  arc A381 (31.8389, 24.257) -> (31.9151, 24.257) centre (31.877, 24.257) ccw
  arc A382 (31.9151, 27.813) -> (31.8389, 27.813) centre (31.877, 27.813) ccw
  line L155 (29.972, 28.321) -> (29.972, 27.94)
  arc A383 (29.9339, 27.94) -> (30.0101, 27.94) centre (29.972, 27.94) ccw
  arc A384 (30.0101, 28.321) -> (29.9339, 28.321) centre (29.972, 28.321) ccw
  line L156 (32.004, 28.321) -> (32.004, 27.94)
  arc A385 (31.9659, 27.94) -> (32.0421, 27.94) centre (32.004, 27.94) ccw
  arc A386 (32.0421, 28.321) -> (31.9659, 28.321) centre (32.004, 28.321) ccw
  line L157 (31.75, 28.575) -> (30.226, 28.575)
  arc A387 (30.226, 28.6131) -> (30.226, 28.5369) centre (30.226, 28.575) ccw
  arc A388 (31.75, 28.5369) -> (31.75, 28.6131) centre (31.75, 28.575) ccw
  arc A389 (22.606, 32.766) -> (22.352, 33.02) centre (22.352, 32.766) ccw
  arc A390 (22.5679, 32.766) -> (22.6441, 32.766) centre (22.606, 32.766) ccw
  arc A391 (22.352, 33.0581) -> (22.352, 32.9819) centre (22.352, 33.02) ccw
  arc A392 (20.828, 33.02) -> (20.574, 32.766) centre (20.828, 32.766) ccw
  arc A393 (20.828, 32.9819) -> (20.828, 33.0581) centre (20.828, 33.02) ccw
  arc A394 (20.5359, 32.766) -> (20.6121, 32.766) centre (20.574, 32.766) ccw
  arc A395 (20.574, 28.194) -> (20.828, 27.94) centre (20.828, 28.194) ccw
  arc A396 (20.6121, 28.194) -> (20.5359, 28.194) centre (20.574, 28.194) ccw
  arc A397 (20.828, 27.9019) -> (20.828, 27.9781) centre (20.828, 27.94) ccw
  arc A398 (22.352, 27.94) -> (22.606, 28.194) centre (22.352, 28.194) ccw
  arc A399 (22.352, 27.9781) -> (22.352, 27.9019) centre (22.352, 27.94) ccw
  arc A400 (22.6441, 28.194) -> (22.5679, 28.194) centre (22.606, 28.194) ccw
  line L158 (20.828, 33.02) -> (22.352, 33.02)
  arc A401 (22.352, 32.9819) -> (22.352, 33.0581) centre (22.352, 33.02) ccw
  arc A402 (20.828, 33.0581) -> (20.828, 32.9819) centre (20.828, 33.02) ccw
  line L159 (22.606, 32.766) -> (22.606, 32.385)
  arc A403 (22.5679, 32.385) -> (22.6441, 32.385) centre (22.606, 32.385) ccw
  arc A404 (22.6441, 32.766) -> (22.5679, 32.766) centre (22.606, 32.766) ccw
  line L160 (22.479, 32.258) -> (22.606, 32.385)
  arc A405 (22.6329, 32.3581) -> (22.5791, 32.4119) centre (22.606, 32.385) ccw
  arc A406 (22.4521, 32.2849) -> (22.5059, 32.2311) centre (22.479, 32.258) ccw
  line L161 (20.574, 32.766) -> (20.574, 32.385)
  arc A407 (20.5359, 32.385) -> (20.6121, 32.385) centre (20.574, 32.385) ccw
  arc A408 (20.6121, 32.766) -> (20.5359, 32.766) centre (20.574, 32.766) ccw
  line L162 (20.701, 32.258) -> (20.574, 32.385)
  arc A409 (20.6009, 32.4119) -> (20.5471, 32.3581) centre (20.574, 32.385) ccw
  arc A410 (20.6741, 32.2311) -> (20.7279, 32.2849) centre (20.701, 32.258) ccw
  line L163 (22.479, 28.702) -> (22.606, 28.575)
  arc A411 (22.5791, 28.5481) -> (22.6329, 28.6019) centre (22.606, 28.575) ccw
  arc A412 (22.5059, 28.7289) -> (22.4521, 28.6751) centre (22.479, 28.702) ccw
  line L164 (22.479, 28.702) -> (22.479, 32.258)
  arc A413 (22.5171, 32.258) -> (22.4409, 32.258) centre (22.479, 32.258) ccw
  arc A414 (22.4409, 28.702) -> (22.5171, 28.702) centre (22.479, 28.702) ccw
  line L165 (20.701, 28.702) -> (20.574, 28.575)
  arc A415 (20.5471, 28.6019) -> (20.6009, 28.5481) centre (20.574, 28.575) ccw
  arc A416 (20.7279, 28.6751) -> (20.6741, 28.7289) centre (20.701, 28.702) ccw
  line L166 (20.701, 28.702) -> (20.701, 32.258)
  arc A417 (20.7391, 32.258) -> (20.6629, 32.258) centre (20.701, 32.258) ccw
  arc A418 (20.6629, 28.702) -> (20.7391, 28.702) centre (20.701, 28.702) ccw
  line L167 (22.606, 28.194) -> (22.606, 28.575)
  arc A419 (22.6441, 28.575) -> (22.5679, 28.575) centre (22.606, 28.575) ccw
  arc A420 (22.5679, 28.194) -> (22.6441, 28.194) centre (22.606, 28.194) ccw
  line L168 (20.574, 28.194) -> (20.574, 28.575)
  arc A421 (20.6121, 28.575) -> (20.5359, 28.575) centre (20.574, 28.575) ccw
  arc A422 (20.5359, 28.194) -> (20.6121, 28.194) centre (20.574, 28.194) ccw
  line L169 (20.828, 27.94) -> (22.352, 27.94)
  arc A423 (22.352, 27.9019) -> (22.352, 27.9781) centre (22.352, 27.94) ccw
  arc A424 (20.828, 27.9781) -> (20.828, 27.9019) centre (20.828, 27.94) ccw
  line L170 (43.18, 27.051) -> (35.56, 27.051)
  arc A425 (35.56, 27.0828) -> (35.56, 27.0193) centre (35.56, 27.0511) ccw
  arc A426 (43.18, 27.0193) -> (43.18, 27.0828) centre (43.18, 27.0511) ccw
  line L171 (35.56, 27.051) -> (35.56, 14.351)
  arc A427 (35.5282, 14.351) -> (35.5918, 14.351) centre (35.56, 14.351) ccw
  arc A428 (35.5918, 27.051) -> (35.5282, 27.051) centre (35.56, 27.051) ccw
  line L172 (35.56, 14.351) -> (43.18, 14.351)
  arc A429 (43.18, 14.3193) -> (43.18, 14.3828) centre (43.18, 14.3511) ccw
  arc A430 (35.56, 14.3828) -> (35.56, 14.3193) centre (35.56, 14.3511) ccw
  line L173 (43.18, 14.351) -> (43.18, 27.051)
  arc A431 (43.2118, 27.051) -> (43.1482, 27.051) centre (43.18, 27.051) ccw
  arc A432 (43.1482, 14.351) -> (43.2118, 14.351) centre (43.18, 14.351) ccw
  line L174 (39.5478, 25.6032) -> (39.9373, 24.4348)
  arc A433 (39.9132, 24.4268) -> (39.9614, 24.4428) centre (39.9373, 24.4348) ccw
  arc A434 (39.5719, 25.6112) -> (39.5237, 25.5952) centre (39.5478, 25.6032) ccw
  line L175 (39.9373, 24.4348) -> (40.3267, 25.6032)
  arc A435 (40.3508, 25.5952) -> (40.3026, 25.6112) centre (40.3267, 25.6032) ccw
  arc A436 (39.9132, 24.4428) -> (39.9614, 24.4268) centre (39.9373, 24.4348) ccw
  line L176 (41.2717, 24.4348) -> (41.012, 24.4348)
  arc A437 (41.012, 24.4602) -> (41.012, 24.4094) centre (41.012, 24.4348) ccw
  arc A438 (41.2717, 24.4094) -> (41.2717, 24.4602) centre (41.2717, 24.4348) ccw
  arc A439 (40.7524, 24.6944) -> (41.012, 24.4348) centre (41.012, 24.6944) ccw
  arc A440 (40.7778, 24.6944) -> (40.727, 24.6944) centre (40.7524, 24.6944) ccw
  arc A441 (41.012, 24.4094) -> (41.012, 24.4602) centre (41.012, 24.4348) ccw
  line L177 (40.7524, 24.6944) -> (40.7524, 25.3436)
  arc A442 (40.7778, 25.3436) -> (40.727, 25.3436) centre (40.7524, 25.3436) ccw
  arc A443 (40.727, 24.6944) -> (40.7778, 24.6944) centre (40.7524, 24.6944) ccw
  arc A444 (41.012, 25.6032) -> (40.7524, 25.3436) centre (41.012, 25.3436) ccw
  arc A445 (41.012, 25.5778) -> (41.012, 25.6286) centre (41.012, 25.6032) ccw
  arc A446 (40.727, 25.3436) -> (40.7778, 25.3436) centre (40.7524, 25.3436) ccw
  line L178 (41.012, 25.6032) -> (41.2717, 25.6032)
  arc A447 (41.2717, 25.5778) -> (41.2717, 25.6286) centre (41.2717, 25.6032) ccw
  arc A448 (41.012, 25.6286) -> (41.012, 25.5778) centre (41.012, 25.6032) ccw
  line L179 (42.2242, 24.4348) -> (41.9645, 24.4348)
  arc A449 (41.9645, 24.4602) -> (41.9645, 24.4094) centre (41.9645, 24.4348) ccw
  arc A450 (42.2242, 24.4094) -> (42.2242, 24.4602) centre (42.2242, 24.4348) ccw
  arc A451 (41.7049, 24.6944) -> (41.9645, 24.4348) centre (41.9645, 24.6944) ccw
  arc A452 (41.7303, 24.6944) -> (41.6795, 24.6944) centre (41.7049, 24.6944) ccw
  arc A453 (41.9645, 24.4094) -> (41.9645, 24.4602) centre (41.9645, 24.4348) ccw
  line L180 (41.7049, 24.6944) -> (41.7049, 25.3436)
  arc A454 (41.7303, 25.3436) -> (41.6795, 25.3436) centre (41.7049, 25.3436) ccw
  arc A455 (41.6795, 24.6944) -> (41.7303, 24.6944) centre (41.7049, 24.6944) ccw
  arc A456 (41.9645, 25.6032) -> (41.7049, 25.3436) centre (41.9645, 25.3436) ccw
  arc A457 (41.9645, 25.5778) -> (41.9645, 25.6286) centre (41.9645, 25.6032) ccw
  arc A458 (41.6795, 25.3436) -> (41.7303, 25.3436) centre (41.7049, 25.3436) ccw
  line L181 (41.9645, 25.6032) -> (42.2242, 25.6032)
  arc A459 (42.2242, 25.5778) -> (42.2242, 25.6286) centre (42.2242, 25.6032) ccw
  arc A460 (41.9645, 25.6286) -> (41.9645, 25.5778) centre (41.9645, 25.6032) ccw
  line L182 (39.6212, 22.0359) -> (39.8159, 22.0359)
  arc A461 (39.8159, 22.0105) -> (39.8159, 22.0613) centre (39.8159, 22.0359) ccw
  arc A462 (39.6212, 22.0613) -> (39.6212, 22.0105) centre (39.6212, 22.0359) ccw
  line L183 (39.8159, 22.0359) -> (39.8159, 21.3868)
  arc A463 (39.7905, 21.3868) -> (39.8413, 21.3868) centre (39.8159, 21.3868) ccw
  arc A464 (39.8413, 22.0359) -> (39.7905, 22.0359) centre (39.8159, 22.0359) ccw
  line L184 (39.8159, 21.3868) -> (39.4264, 21.3868)
  arc A465 (39.4264, 21.4122) -> (39.4264, 21.3614) centre (39.4264, 21.3868) ccw
  line L185 (24.765, 30.48) -> (28.575, 30.48)
  arc A466 (28.575, 30.4292) -> (28.575, 30.5308) centre (28.575, 30.48) ccw
  arc A467 (24.765, 30.5308) -> (24.765, 30.4292) centre (24.765, 30.48) ccw
  line L186 (38.735, 35.56) -> (34.925, 35.56)
  arc A468 (34.925, 35.6108) -> (34.925, 35.5092) centre (34.925, 35.56) ccw
  arc A469 (38.735, 35.5092) -> (38.735, 35.6108) centre (38.735, 35.56) ccw
  line L187 (31.8403, 15.0932) -> (32.0873, 15.2908)
  arc A470 (32.1031, 15.271) -> (32.0714, 15.3106) centre (32.0872, 15.2908) ccw
  arc A471 (31.8244, 15.1131) -> (31.8562, 15.0734) centre (31.8403, 15.0933) ccw
  line L188 (32.0873, 15.2908) -> (32.0873, 14.4018)
  arc A472 (32.0619, 14.4018) -> (32.1127, 14.4018) centre (32.0873, 14.4018) ccw
  line L189 (30.607, 32.6025) -> (30.1244, 32.6025)
  arc A473 (30.1244, 32.6342) -> (30.1244, 32.5707) centre (30.1244, 32.6025) ccw
  arc A474 (30.607, 32.5707) -> (30.607, 32.6342) centre (30.607, 32.6025) ccw
  line L190 (30.1244, 32.6025) -> (30.1244, 32.7365)
  arc A475 (30.1562, 32.7365) -> (30.0927, 32.7365) centre (30.1244, 32.7365) ccw
  arc A476 (30.0927, 32.6025) -> (30.1562, 32.6025) centre (30.1244, 32.6025) ccw
  arc A477 (30.2585, 32.8706) -> (30.1244, 32.7365) centre (30.2585, 32.7365) ccw
  arc A478 (30.2585, 32.8388) -> (30.2585, 32.9023) centre (30.2585, 32.8705) ccw
  arc A479 (30.0927, 32.7365) -> (30.1562, 32.7365) centre (30.1244, 32.7365) ccw
  line L191 (30.2585, 32.8706) -> (30.4729, 32.8706)
  arc A480 (30.4729, 32.8388) -> (30.4729, 32.9023) centre (30.4729, 32.8705) ccw
  arc A481 (30.2585, 32.9023) -> (30.2585, 32.8388) centre (30.2585, 32.8705) ccw
  arc A482 (30.607, 32.7365) -> (30.4729, 32.8706) centre (30.4729, 32.7365) ccw
  arc A483 (30.5753, 32.7365) -> (30.6387, 32.7365) centre (30.607, 32.7365) ccw
  arc A484 (30.4729, 32.9023) -> (30.4729, 32.8388) centre (30.4729, 32.8705) ccw
  line L192 (30.607, 32.7365) -> (30.607, 32.6025)
  arc A485 (30.5753, 32.6025) -> (30.6388, 32.6025) centre (30.6071, 32.6025) ccw
  arc A486 (30.6388, 32.7365) -> (30.5753, 32.7365) centre (30.6071, 32.7365) ccw
  line L193 (30.2316, 33.1694) -> (30.1244, 33.3035)
  arc A487 (30.1492, 33.3233) -> (30.0996, 33.2836) centre (30.1244, 33.3034) ccw
  arc A488 (30.2069, 33.1496) -> (30.2564, 33.1892) centre (30.2317, 33.1694) ccw
  line L194 (30.1244, 33.3035) -> (30.607, 33.3035)
  arc A489 (30.607, 33.2717) -> (30.607, 33.3352) centre (30.607, 33.3034) ccw
  arc A490 (30.1244, 33.3352) -> (30.1244, 33.2717) centre (30.1244, 33.3034) ccw
  line L195 (30.607, 33.1694) -> (30.607, 33.4375)
  arc A491 (30.6388, 33.4375) -> (30.5753, 33.4375) centre (30.6071, 33.4375) ccw
  arc A492 (30.5753, 33.1694) -> (30.6388, 33.1694) centre (30.6071, 33.1694) ccw
  arc A493 (32.1127, 15.2908) -> (32.0619, 15.2908) centre (32.0873, 15.2908) ccw
  line L196 (31.8403, 14.4018) -> (32.3342, 14.4018)
  arc A494 (32.3342, 14.3764) -> (32.3342, 14.4272) centre (32.3342, 14.4018) ccw
  arc A495 (27.3558, 21.0707) -> (27.3558, 21.0199) centre (27.3558, 21.0453) ccw
  arc A496 (31.8403, 14.4272) -> (31.8403, 14.3764) centre (31.8403, 14.4018) ccw
  line L197 (29.2467, 23.7927) -> (29.2467, 23.5458)
  arc A497 (28.7274, 23.7927) -> (28.7782, 23.7927) centre (28.7528, 23.7927) ccw
  line L198 (27.3558, 20.6502) -> (27.3558, 21.5392)
  line L199 (33.3756, 32.6025) -> (32.893, 32.6025)
  arc A498 (32.893, 32.6342) -> (32.893, 32.5707) centre (32.893, 32.6025) ccw
  arc A499 (33.3756, 32.5707) -> (33.3756, 32.6342) centre (33.3756, 32.6025) ccw
  line L200 (32.893, 32.6025) -> (32.893, 32.7365)
  arc A500 (32.9248, 32.7365) -> (32.8612, 32.7365) centre (32.893, 32.7365) ccw
  arc A501 (32.8612, 32.6025) -> (32.9248, 32.6025) centre (32.893, 32.6025) ccw
  arc A502 (33.0271, 32.8706) -> (32.893, 32.7365) centre (33.0271, 32.7365) ccw
  arc A503 (33.0271, 32.8388) -> (33.0271, 32.9023) centre (33.0271, 32.8705) ccw
  arc A504 (32.8612, 32.7365) -> (32.9248, 32.7365) centre (32.893, 32.7365) ccw
  line L201 (33.0271, 32.8706) -> (33.2415, 32.8706)
  arc A505 (33.2415, 32.8388) -> (33.2415, 32.9023) centre (33.2415, 32.8705) ccw